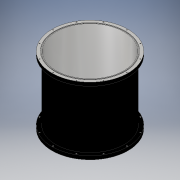
# Autodesk Inventor part: vacuum jacket
Saved by Autodesk Inventor 2018 (Build 220112000, 112)
## iProperties
Created: 2018-09-07
Part Number: vacuum jacket
Material: Generic
Document SubType Name: Modeling
Designer: freyja
Density: 1 g/cm^3
Appearance: Aluminum - Dark
Author: freyja
Autodesk Inventor part; units mm, degrees
ref_plane "YZ Plane" through (0, 0, 0) normal (1, 0, 0) x (0, 1, 0)
ref_plane "XZ Plane" through (0, 0, 0) normal (0, 1, 0) x (-1, 0, 0)
ref_plane "XY Plane" through (0, 0, 0) normal (0, 0, 1) x (1, 0, 0)
sketch "Sketch1" plane through (0, 0, 0) normal (0, 1, 0) x (-1, 0, 0)
  circle A0 centre (0, 0) radius 273.05
  circle A1 centre (0, 0) radius 242.8875
  dimension "d0" = 546.1
  dimension "d1" = 485.775
  constraints: 2 centre point, 2 coincident
  measures "d0" diameter of A0
  measures "d1" diameter of A1
extrude "Extrusion1" add sketch "Sketch1" along normal blind 25.4
sketch "Sketch2" plane through (0, 25.4, 0) normal (0, 1, 0) x (1, 0, 0)
  circle A0 centre (0, 0) radius 247.65
  circle A1 centre (0, 0) radius 252.4125
  dimension "d4" = 495.3
  dimension "d5" = 504.825
  constraints: 2 centre point, 2 coincident
  measures "d4" diameter of A0
  measures "d5" diameter of A1
extrude "Extrusion2" cut sketch "Sketch2" against normal blind 3.175
sketch "Sketch3" plane through (0, 25.4, 0) normal (0, 1, 0) x (1, 0, 0)
  line L0 (0, 0) -> (-265.25, 0) construction
  dimension "d8" = 265.25
  constraints: 2 end point, 1 horizontal
  measures "d8" distance of L0.start L0.end
hole "Hole1" at (-265.25, 25.4, 0) direction (0, -1, 0) diameter 6.1976 end up to face face through (3.6324, 0, -262.7503) facing (0, -1, 0)
pattern_circular "Circular Pattern1" count 12 over 360 about axis through (0, -10, 0) along (0, 1, 0) of "Hole1"
sketch "Sketch4" plane through (0, 0, 0) normal (0, -1, 0) x (1, 0, 0)
  circle A0 centre (0, 0) radius 242.8875
  circle A1 centre (0, 0) radius 246.0625
  dimension "d19" = 485.775
  dimension "d20" = 492.125
  constraints: 2 centre point, 2 coincident
  measures "d19" diameter of A0
  measures "d20" diameter of A1
extrude "Extrusion3" add sketch "Sketch4" along normal blind 431.8
sketch "Sketch5" plane through (0, -431.8, 0) normal (0, -1, 0) x (1, 0, 0)
  circle A0 centre (0, 0) radius 273.05
  circle A1 centre (0, 0) radius 242.8875
  dimension "d24" = 546.1
  dimension "d23" = 485.775
  constraints: 2 centre point, 2 coincident
  measures "d24" diameter of A0
  measures "d23" diameter of A1
extrude "Extrusion4" add sketch "Sketch5" along normal blind 25.4
sketch "Sketch7" plane through (0, -457.2, 0) normal (0, -1, 0) x (-1, 0, 0)
  line L0 (0, 0) -> (-265.25, 0) construction
  dimension "d34" = 265.25
  constraints: 2 end point, 1 horizontal
  measures "d34" distance of L0.start L0.end
hole "Hole2" at (265.25, -457.2, 0) direction (0, 1, 0) diameter 8.9916 end up to face face through (-3.6799, -431.8, -263.8076) facing (0, 1, 0) clearance for "Hex Head Cap Screw" size "M8" standard "Ansi Metric M Profile"
pattern_circular "Circular Pattern2" count 12 over 360 about axis through (0, 0, 0) along (0, -1, 0) of "Hole2"
body "Solid1"
